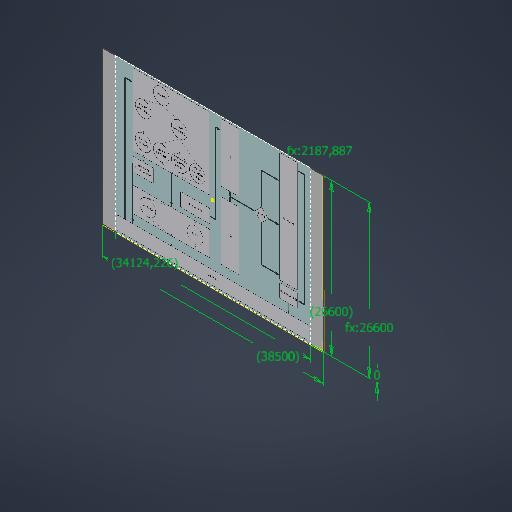
# Autodesk Inventor part: Floor
Saved by Autodesk Inventor 2026.2 (Build 302298000, 298)
## iProperties
Created: 2025-11-24
Part Number: Floor
Material: Genérico
Document SubType Name: Modeling
Designer: USUARIO
Density: 1 g/cm^3
Appearance: Valor por defecto
Author: USUARIO
Autodesk Inventor part; units mm, degrees
ref_plane "YZ Plane" through (0, 0, 0) normal (1, 0, 0) x (0, 1, 0)
ref_plane "XZ Plane" through (0, 0, 0) normal (0, 1, 0) x (-1, 0, 0)
ref_plane "XY Plane" through (0, 0, 0) normal (0, 0, 1) x (1, 0, 0)
sketch "Boceto1" plane through (0, 0, 0) normal (0, 0, 1) x (1, 0, 0)
  line L0 (-19250, 13300) -> (19250, 13300)
  line L1 (19250, 13300) -> (19250, -13300)
  line L2 (19250, -13300) -> (-19250, -13300)
  line L3 (-19250, -13300) -> (-19250, 13300)
  point P0 (0, 0)
  dimension "d0" = 38500
  dimension "d1" = 26600
  dimension "d2" = 19250
  dimension "d3" = 13300
  constraints: 8 end point, 2 parallel, 1 horizontal, 1 perpendicular
  measures "d0" distance of L0.start L0.end
  measures "d1" distance of L2.end L0.start
  measures "d2" distance from line of L3 point (0, 0)
  measures "d3" distance from line of L0 point (0, 0)
extrude "Extrusión1" add sketch "Boceto1" along normal blind 100
sketch "Boceto2" plane through (0, 0, 100) normal (0, 0, 1) x (1, 0, 0)
  line L0 (17062.1132, -13300) -> (-17062.1132, -13300) construction
  line L1 (-17062.1132, -13300) -> (-17062.1132, 13300) construction
  line L2 (-17062.1132, 13300) -> (17062.1132, 13300) construction
  line L3 (17062.1132, 13300) -> (17062.1132, -13300) construction
  line L4 (-19250, -13300) -> (19250, -13300) projected
  line L5 (19250, -13300) -> (19250, 13300) projected
  point P0 (0, 0)
  dimension "d21" = 26600
  dimension "d22" = 26600
  dimension "d24" = 0
  dimension "d25" = 2187.8868
  dimension "d26" = 34124.2264
  dimension "d27" = 38500
  constraints: 1 collinear, 2 other
  measures "d21" distance of L4.end L5.end
  measures "d22" distance of L2.end L0.start
  measures "d24" distance between parallel lines of L0 L4
  measures "d25" distance between parallel lines of L5 L3
  measures "d26" distance of L0.start L0.end
  measures "d27" distance of L4.start L4.end
equation "\"d2\" = 0.5 * d0"
equation "\"d3\" = 0.5 * d1"
equation "\"d22\" = d21"
equation "\"d25\" = -0.5 * d26 + 0.5 * d27"
